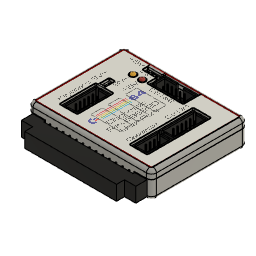
Diag_UP_PCB_v3_noVM v12 (Autodesk Fusion 360 design; units mm, degrees)
Autodesk Fusion 360 part; units mm, degrees
(part 1 of 2)
sketch "C64_Userport_Test" plane through (0, 0, 0) normal (0, 0, 1) x (1, 0, 0)
  line L0 (15.7163, 51.435) -> (15.7163, 52.705)
  line L1 (8.7313, 50.8) -> (8.0962, 51.435)
  line L2 (15.0813, 50.8) -> (15.7163, 51.435)
  line L3 (8.0962, 52.705) -> (8.7313, 53.34)
  line L4 (10.6363, 51.435) -> (10.0013, 50.8)
  line L5 (15.0813, 50.8) -> (13.8113, 50.8)
  line L6 (12.5412, 50.8) -> (11.2713, 50.8)
  line L7 (13.8113, 50.8) -> (13.1763, 51.435)
  line L8 (13.8113, 53.34) -> (15.0813, 53.34)
  line L9 (3.175, 30.6388) -> (2.54, 31.2738)
  line L10 (2.54, 33.8137) -> (2.54, 35.0838)
  line L11 (3.175, 33.1788) -> (2.54, 33.8137)
  line L12 (10.6363, 52.705) -> (11.2713, 53.34)
  line L13 (5.08, 32.5438) -> (5.08, 31.2738)
  arc A0 (8.3, 43.5) -> (8.3, 46.5) centre (7.5, 45) ccw
  line L14 (5.08, 35.0838) -> (5.08, 33.8137)
  line L15 (3.175, 35.7188) -> (2.54, 35.7188)
  line L16 (2.54, 31.2738) -> (2.54, 32.5438)
  arc A1 (6.7, 46.5) -> (6.7, 43.5) centre (7.5, 45) ccw
  arc A2 (6.7, 46.5) -> (6.7, 43.5) centre (7.5, 45) ccw
  line L17 (10.6363, 51.435) -> (10.6363, 52.705)
  line L18 (12.5412, 53.34) -> (13.1763, 52.705)
  line L19 (8.7313, 53.34) -> (10.0013, 53.34)
  line L20 (4.445, 30.6388) -> (3.175, 30.6388)
  line L21 (5.08, 35.0838) -> (4.445, 35.7188)
  line L22 (10.0013, 53.34) -> (10.6363, 52.705)
  line L23 (4.445, 33.1788) -> (3.175, 33.1788)
  line L24 (15.7163, 52.705) -> (15.7163, 53.34)
  line L25 (13.1763, 52.705) -> (13.8113, 53.34)
  line L26 (13.1763, 51.435) -> (12.5412, 50.8)
  line L27 (11.2713, 53.34) -> (12.5412, 53.34)
  line L28 (8.0962, 51.435) -> (8.0962, 52.705)
  line L29 (15.7163, 53.34) -> (15.0813, 53.34)
  line L30 (4.445, 33.1788) -> (5.08, 32.5438)
  line L31 (2.54, 35.7188) -> (2.54, 35.0838)
  line L32 (11.2713, 50.8) -> (10.6363, 51.435)
  line L33 (10.0013, 50.8) -> (8.7313, 50.8)
  line L34 (2.54, 32.5438) -> (3.175, 33.1788)
  arc A3 (13.8, 43.5) -> (13.8, 46.5) centre (13, 45) ccw
  arc A4 (13.8, 43.5) -> (13.8, 46.5) centre (13, 45) ccw
  arc A5 (8.3, 43.5) -> (8.3, 46.5) centre (7.5, 45) ccw
  line L35 (5.08, 31.2738) -> (4.445, 30.6388)
  line L36 (4.445, 35.7188) -> (3.175, 35.7188)
  line L37 (5.08, 33.8137) -> (4.445, 33.1788)
  line L38 (13.1763, 51.435) -> (13.1763, 52.705)
  arc A6 (12.2, 46.5) -> (12.2, 43.5) centre (13, 45) ccw
  arc A7 (12.2, 46.5) -> (12.2, 43.5) centre (13, 45) ccw
  arc A8 (15.9068, 14.224) -> (15.9068, 16.256) centre (15.9068, 15.24) ccw
  arc A9 (15.9068, 34.8615) -> (15.9068, 36.8935) centre (15.9068, 35.8775) ccw
  line L39 (32.6707, 38.7985) -> (32.6707, 32.9565)
  line L40 (15.9068, 32.9565) -> (15.9068, 34.8615)
  line L41 (32.6707, 18.161) -> (32.6707, 12.319)
  arc A10 (15.9068, 24.5427) -> (15.9068, 26.5747) centre (15.9068, 25.5587) ccw
  line L42 (32.6707, 38.7985) -> (15.9068, 38.7985)
  line L43 (15.9068, 18.161) -> (15.9068, 16.256)
  line L44 (15.9068, 32.9565) -> (32.6707, 32.9565)
  line L45 (15.9068, 22.6378) -> (15.9068, 24.5428)
  line L46 (32.6707, 28.4798) -> (32.6707, 22.6378)
  line L47 (15.9068, 28.4798) -> (15.9068, 26.5748)
  line L48 (15.9068, 22.6378) -> (32.6707, 22.6378)
  line L49 (15.9068, 12.319) -> (15.9068, 14.224)
  line L50 (15.9068, 12.319) -> (32.6707, 12.319)
  line L51 (15.9068, 38.7985) -> (15.9068, 36.8935)
  line L52 (32.6707, 28.4798) -> (15.9068, 28.4798)
  line L53 (32.6707, 18.161) -> (15.9068, 18.161)
  line L54 (9.6203, 51.816) -> (9.6203, 52.324)
  arc A11 (6.7, 43.5) -> (8.3, 43.5) centre (7.5, 45) ccw
  line L55 (11.6523, 51.816) -> (12.1603, 51.816)
  line L56 (4.064, 34.7028) -> (3.556, 34.7028)
  line L57 (14.1923, 51.816) -> (14.7003, 51.816)
  line L58 (9.1123, 51.816) -> (9.6203, 51.816)
  line L59 (4.064, 32.1628) -> (3.556, 32.1628)
  line L60 (12.1603, 52.324) -> (11.6523, 52.324)
  line L61 (4.064, 34.1948) -> (4.064, 34.7028)
  line L62 (3.556, 34.7028) -> (3.556, 34.1948)
  line L63 (14.7003, 52.324) -> (14.1923, 52.324)
  line L64 (3.556, 31.6548) -> (4.064, 31.6548)
  line L65 (14.1923, 52.324) -> (14.1923, 51.816)
  line L66 (14.7003, 51.816) -> (14.7003, 52.324)
  line L67 (3.556, 32.1628) -> (3.556, 31.6548)
  line L68 (3.556, 34.1948) -> (4.064, 34.1948)
  line L69 (9.1123, 52.324) -> (9.1123, 51.816)
  circle A12 centre (7.5, 45) radius 1.5
  line L70 (12.1603, 51.816) -> (12.1603, 52.324)
  line L71 (9.6203, 52.324) -> (9.1123, 52.324)
  line L72 (6.7, 46.5) -> (8.3, 46.5)
  line L73 (12.2, 46.5) -> (13.8, 46.5)
  line L74 (4.064, 31.6548) -> (4.064, 32.1628)
  line L75 (11.6523, 52.324) -> (11.6523, 51.816)
  arc A13 (12.2, 43.5) -> (13.8, 43.5) centre (13, 45) ccw
  circle A14 centre (13, 45) radius 1.5
sketch "DXF import" plane through (0, 0, 0) normal (0, 0, 1) x (1, 0, 0) in component "PCB"
  arc A0 (0, 1) -> (1, 0) centre (1, 1) ccw
  line L0 (53, 1) -> (53, 54)
  line L1 (0, 1) -> (0, 54)
  arc A1 (53, 54) -> (52, 55) centre (52, 54) ccw
  line L2 (52, 55) -> (1, 55)
  line L3 (1, 0) -> (52, 0)
  arc A2 (1, 55) -> (0, 54) centre (1, 54) ccw
  arc A3 (52, 0) -> (53, 1) centre (52, 1) ccw
  circle A4 centre (4, 51) radius 3.1
  line L4 (32.6707, 38.7985) -> (32.6707, 32.9565)
  arc A5 (15.9068, 24.5428) -> (15.9068, 26.5748) centre (15.9068, 25.5588) ccw
  line L5 (15.9068, 28.4798) -> (15.9068, 26.5748)
  line L6 (15.9068, 32.9565) -> (32.6707, 32.9565)
  line L7 (15.9068, 22.6378) -> (15.9068, 24.5428)
  line L8 (15.9068, 22.6378) -> (32.6707, 22.6378)
  line L9 (32.6707, 28.4798) -> (32.6707, 22.6378)
  line L10 (32.6707, 28.4798) -> (15.9068, 28.4798)
  line L11 (50.18, 0) -> (50.18, -1)
  line L12 (32.6707, 38.7985) -> (15.9068, 38.7985)
  circle A6 centre (49, 51) radius 3.1
  line L13 (15.9068, 18.161) -> (15.9068, 16.256)
  line L14 (46.72, -1) -> (46.72, 0)
  line L15 (15.9068, 12.319) -> (15.9068, 14.224)
  circle A7 centre (49, 51) radius 1.5875
  line L16 (46.72, 0) -> (46.22, 0)
  line L17 (32.6707, 18.161) -> (15.9068, 18.161)
  arc A8 (15.9068, 14.224) -> (15.9068, 16.256) centre (15.9068, 15.24) ccw
  line L18 (15.9068, 12.319) -> (32.6707, 12.319)
  line L19 (32.6707, 18.161) -> (32.6707, 12.319)
  line L20 (49.45, 0.1) -> (49.45, -1)
  line L21 (47.45, 0.1) -> (47.45, -1)
  line L22 (46.22, 0) -> (46.22, -1)
  line L23 (50.68, -1) -> (50.68, 0)
  arc A9 (15.9068, 34.8615) -> (15.9068, 36.8935) centre (15.9068, 35.8775) ccw
  line L24 (50.68, 0) -> (50.18, 0)
  line L25 (31.61, 0.1) -> (31.61, -1)
  line L26 (15.9068, 38.7985) -> (15.9068, 36.8935)
  circle A10 centre (4, 51) radius 1.5875
  line L27 (15.9068, 32.9565) -> (15.9068, 34.8615)
  line L28 (22.96, 0) -> (22.46, 0)
  line L29 (7.85, 0.1) -> (7.85, -1)
  line L30 (42.76, -1) -> (42.76, 0)
  line L31 (43.49, 0.1) -> (43.49, -1)
  line L32 (45.49, 0.1) -> (45.49, -1)
  line L33 (30.88, -1) -> (30.88, 0)
  line L34 (7.12, -1) -> (7.12, 0)
  line L35 (22.46, 0) -> (22.46, -1)
  line L36 (7.12, 0) -> (6.62, 0)
  line L37 (35.57, 0.1) -> (35.57, -1)
  line L38 (6.62, 0) -> (6.62, -1)
  line L39 (14.54, 0) -> (14.54, -1)
  line L40 (37.57, 0.1) -> (37.57, -1)
  line L41 (38.8, -1) -> (38.8, 0)
  line L42 (15.04, 0) -> (14.54, 0)
  line L43 (18.5, 0) -> (18.5, -1)
  line L44 (29.65, 0.1) -> (29.65, -1)
  line L45 (30.88, 0) -> (30.38, 0)
  line L46 (27.65, 0.1) -> (27.65, -1)
  line L47 (26.42, 0) -> (26.42, -1)
  line L48 (38.8, 0) -> (38.3, 0)
  line L49 (34.84, 0) -> (34.34, 0)
  line L50 (39.53, 0.1) -> (39.53, -1)
  line L51 (42.26, 0) -> (42.26, -1)
  line L52 (42.76, 0) -> (42.26, 0)
  line L53 (26.92, -1) -> (26.92, 0)
  line L54 (38.3, 0) -> (38.3, -1)
  line L55 (33.61, 0.1) -> (33.61, -1)
  line L56 (34.34, 0) -> (34.34, -1)
  line L57 (26.92, 0) -> (26.42, 0)
  line L58 (30.38, 0) -> (30.38, -1)
  line L59 (34.84, -1) -> (34.84, 0)
  line L60 (41.53, 0.1) -> (41.53, -1)
  line L61 (21.73, 0.1) -> (21.73, -1)
  line L62 (15.77, 0.1) -> (15.77, -1)
  line L63 (11.08, -1) -> (11.08, 0)
  line L64 (23.69, 0.1) -> (23.69, -1)
  line L65 (19.73, 0.1) -> (19.73, -1)
  line L66 (25.69, 0.1) -> (25.69, -1)
  line L67 (19, -1) -> (19, 0)
  line L68 (11.81, 0.1) -> (11.81, -1)
  line L69 (54.17, -6.8) -> (54.17, -11.6)
  line L70 (11.08, 0) -> (10.58, 0)
  line L71 (22.96, -1) -> (22.96, 0)
  line L72 (55.97, -6.8) -> (54.17, -6.8)
  line L73 (-6.03, -6.8) -> (-7.58, -6.8)
  line L74 (59.37, -6.8) -> (55.97, -6.8)
  line L75 (60.92, -6.8) -> (59.37, -6.8)
  line L76 (19, 0) -> (18.5, 0)
  line L77 (9.85, 0.1) -> (9.85, -1)
  line L78 (53.47, 0) -> (53.47, -1)
  line L79 (3.16, -1) -> (3.16, 0)
  line L80 (17.77, 0.1) -> (17.77, -1)
  line L81 (-2.63, -6.8) -> (-2.63, -5.2)
  line L82 (-4.33, 0) -> (-4.33, -2.8667)
  line L83 (57.67, -3.6853) -> (57.67, -3.548)
  line L84 (55.97, -4.2) -> (55.97, -2.6)
  line L85 (59.37, -1.6) -> (59.37, 0)
  line L86 (60.92, 0) -> (59.37, 0)
  line L87 (59.37, 0) -> (57.67, 0)
  line L88 (-4.33, -3.548) -> (-4.33, -3.6853)
  line L89 (-4.33, -4.3667) -> (-4.33, -7.2333)
  line L90 (55.97, -1.6) -> (55.97, 0)
  line L91 (57.67, 0) -> (55.97, 0)
  line L92 (-0.83, -6.8) -> (-2.63, -6.8)
  line L93 (-2.63, -4.2) -> (-2.63, -2.6)
  line L94 (-4.33, -8.7333) -> (-4.33, -11.6)
  line L95 (-4.33, 0) -> (-6.03, 0)
  line L96 (10.58, 0) -> (10.58, -1)
  line L97 (13.81, 0.1) -> (13.81, -1)
  line L98 (5.89, 0.1) -> (5.89, -1)
  line L99 (-2.63, -1.6) -> (-2.63, 0)
  line L100 (-6.03, -1.6) -> (-6.03, 0)
  line L101 (55.97, 0) -> (53.47, 0)
  line L102 (-7.58, 0) -> (-7.58, -6.8)
  line L103 (3.16, 0) -> (2.66, 0)
  line L104 (3.89, 0.1) -> (3.89, -1)
  line L105 (15.04, -1) -> (15.04, 0)
  line L106 (59.37, -4.2) -> (59.37, -2.6)
  line L107 (-6.03, -6.8) -> (-6.03, -5.2)
  line L108 (2.66, 0) -> (2.66, -1)
  line L109 (51.81, 14.73) -> (52.6038, 14.73)
  line L110 (52.6038, 23.62) -> (52.6038, 17.27)
  line L111 (-0.13, 0) -> (-2.63, 0)
  line L112 (60.92, 0) -> (60.92, -6.8)
  line L113 (46.2537, 8.38) -> (44.825, 8.38)
  line L114 (51.81, 17.27) -> (52.6038, 17.27)
  line L115 (-0.83, -11.6) -> (-0.83, -6.8)
  line L116 (-6.03, 0) -> (-7.58, 0)
  line L117 (57.67, -2.8667) -> (57.67, 0)
  line L118 (51.3338, 17.27) -> (51.81, 17.27)
  line L119 (46.2537, 23.62) -> (52.6038, 23.62)
  line L120 (44.6662, 22.35) -> (44.825, 22.35)
  line L121 (51.3338, 9.65) -> (46.2537, 9.65)
  line L122 (44.825, 22.35) -> (44.825, 22.8263)
  line L123 (57.67, -11.6) -> (57.67, -8.7333)
  line L124 (43.3962, 23.62) -> (44.825, 23.62)
  line L125 (51.81, 14.73) -> (51.81, 9.1737)
  line L126 (46.2537, 22.35) -> (46.2537, 22.8263)
  line L127 (57.67, -7.2333) -> (57.67, -4.3667)
  line L128 (44.825, 8.38) -> (43.3962, 8.38)
  line L129 (51.3338, 22.35) -> (51.3338, 17.27)
  line L130 (44.825, 9.65) -> (44.825, 9.1737)
  line L131 (55.97, -6.8) -> (55.97, -5.2)
  line L132 (51.3338, 22.35) -> (51.81, 22.8263)
  line L133 (51.3338, 14.73) -> (51.3338, 9.65)
  line L134 (-4.33, -7.9147) -> (-4.33, -8.052)
  line L135 (53.47, -1) -> (-0.13, -1)
  line L136 (-2.63, -6.8) -> (-6.03, -6.8)
  line L137 (44.6662, 9.65) -> (44.6662, 22.35)
  line L138 (46.2537, 22.35) -> (51.3338, 22.35)
  line L139 (54.17, -11.6) -> (-0.83, -11.6)
  line L140 (57.67, -8.052) -> (57.67, -7.9147)
  line L141 (52.6038, 14.73) -> (52.6038, 8.38)
  line L142 (51.3338, 17.27) -> (51.3338, 14.73)
  line L143 (43.3962, 8.38) -> (43.3962, 23.62)
  line L144 (46.2537, 9.65) -> (44.825, 9.65)
  line L145 (51.3338, 14.73) -> (51.81, 14.73)
  line L146 (-6.03, -4.2) -> (-6.03, -2.6)
  line L147 (52.6038, 17.27) -> (52.6038, 14.73)
  line L148 (52.6038, 8.38) -> (46.2537, 8.38)
  line L149 (44.825, 9.65) -> (44.6662, 9.65)
  line L150 (59.37, -6.8) -> (59.37, -5.2)
  line L151 (44.825, 23.62) -> (46.2537, 23.62)
  line L152 (44.825, 22.35) -> (46.2537, 22.35)
  line L153 (-2.63, 0) -> (-4.33, 0)
  line L154 (-0.13, -1) -> (-0.13, 0)
  arc A11 (43.3962, 35.4763) -> (43.3962, 34.3651) centre (43.3962, 34.9207) ccw
  line L155 (46.2537, 9.1737) -> (51.81, 9.1737)
  line L156 (44.19, 9.1737) -> (44.6662, 9.65)
  arc A12 (43.3962, 10.92) -> (43.3962, 9.65) centre (43.3962, 10.285) ccw
  line L157 (44.825, 22.8263) -> (44.19, 22.8263)
  arc A13 (43.3962, 27.38) -> (43.3962, 26.11) centre (43.3962, 26.745) ccw
  line L158 (44.825, 24.84) -> (43.3962, 24.84)
  line L159 (44.825, 25.6337) -> (44.825, 24.84)
  line L160 (51.81, 25.6337) -> (51.3338, 26.11)
  arc A14 (43.3962, 22.35) -> (43.3962, 21.08) centre (43.3962, 21.715) ccw
  line L161 (44.19, 25.6337) -> (44.825, 25.6337)
  line L162 (44.6662, 26.11) -> (44.6662, 43.89)
  line L163 (44.825, 26.11) -> (44.6662, 26.11)
  line L164 (43.3962, 45.16) -> (44.825, 45.16)
  line L165 (46.2537, 44.3663) -> (46.2537, 45.16)
  line L166 (44.825, 43.89) -> (44.825, 44.3663)
  line L167 (51.81, 9.1737) -> (51.3338, 9.65)
  arc A15 (43.3962, 16.4763) -> (43.3962, 15.3651) centre (43.3962, 15.9207) ccw
  line L168 (46.2537, 22.8263) -> (46.2537, 23.62)
  line L169 (44.19, 9.1737) -> (44.825, 9.1737)
  line L170 (44.825, 9.1737) -> (44.825, 8.38)
  line L171 (51.81, 17.27) -> (51.81, 22.8263)
  line L172 (46.2537, 9.65) -> (46.2537, 9.1737)
  line L173 (46.2537, 22.8263) -> (51.81, 22.8263)
  line L174 (44.6662, 22.35) -> (44.19, 22.8263)
  line L175 (51.3338, 37.0638) -> (51.3338, 32.9362)
  line L176 (51.3338, 37.0638) -> (51.81, 37.0638)
  line L177 (44.825, 44.3663) -> (44.19, 44.3663)
  line L178 (51.3338, 43.89) -> (51.81, 44.3663)
  line L179 (44.825, 43.89) -> (46.2537, 43.89)
  line L180 (46.2537, 25.6337) -> (46.2537, 24.84)
  line L181 (51.3338, 43.89) -> (51.3338, 37.0638)
  line L182 (46.2537, 43.89) -> (46.2537, 44.3663)
  line L183 (51.81, 32.9362) -> (52.6038, 32.9362)
  line L184 (51.3338, 26.11) -> (46.2537, 26.11)
  line L185 (46.2537, 9.1737) -> (46.2537, 8.38)
  line L186 (44.19, 25.6337) -> (44.19, 44.3663)
  line L187 (44.19, 9.1737) -> (44.19, 22.8263)
  line L188 (46.2537, 25.6337) -> (51.81, 25.6337)
  line L189 (44.19, 25.6337) -> (44.6662, 26.11)
  line L190 (44.825, 22.8263) -> (44.825, 23.62)
  line L191 (51.81, 32.9362) -> (51.81, 25.6337)
  line L192 (44.6662, 43.89) -> (44.825, 43.89)
  arc A16 (43.3962, 43.89) -> (43.3962, 42.62) centre (43.3962, 43.255) ccw
  line L193 (44.825, 26.11) -> (44.825, 25.6337)
  line L194 (52.6038, 37.0638) -> (52.6038, 32.9362)
  line L195 (43.3962, 24.84) -> (43.3962, 45.16)
  line L196 (46.2537, 26.11) -> (44.825, 26.11)
  line L197 (44.825, 44.3663) -> (44.825, 45.16)
  line L198 (37.16, 46.825) -> (37.16, 45.3962)
  line L199 (18.11, 48.2537) -> (17.6337, 48.2537)
  line L200 (37.16, 54.6038) -> (37.16, 48.2537)
  arc A17 (26.5238, 45.3962) -> (27.635, 45.3962) centre (27.0794, 45.3962) ccw
  line L201 (51.3338, 32.9362) -> (51.3338, 26.11)
  line L202 (36.3663, 46.19) -> (36.3663, 46.825)
  line L203 (51.81, 37.0638) -> (51.81, 44.3663)
  line L204 (29.0638, 53.81) -> (29.0638, 54.6038)
  line L205 (29.0638, 53.3338) -> (35.89, 53.3338)
  line L206 (46.2537, 45.16) -> (52.6038, 45.16)
  line L207 (17.6337, 46.825) -> (16.84, 46.825)
  line L208 (37.16, 48.2537) -> (37.16, 46.825)
  line L209 (46.2537, 43.89) -> (51.3338, 43.89)
  line L210 (52.6038, 32.9362) -> (52.6038, 24.84)
  line L211 (18.11, 53.3338) -> (24.9362, 53.3338)
  line L212 (36.3663, 48.2537) -> (36.3663, 53.81)
  line L213 (52.6038, 45.16) -> (52.6038, 37.0638)
  line L214 (51.3338, 32.9362) -> (51.81, 32.9362)
  line L215 (44.6662, 43.89) -> (44.19, 44.3663)
  line L216 (17.6337, 46.825) -> (17.6337, 46.19)
  line L217 (18.11, 46.6662) -> (18.11, 46.825)
  line L218 (52.6038, 24.84) -> (46.2537, 24.84)
  line L219 (18.11, 46.825) -> (18.11, 48.2537)
  line L220 (24.9362, 53.81) -> (24.9362, 54.6038)
  line L221 (29.0638, 54.6038) -> (37.16, 54.6038)
  line L222 (29.0638, 53.3338) -> (29.0638, 53.81)
  line L223 (18.11, 46.825) -> (17.6337, 46.825)
  line L224 (36.3663, 46.19) -> (17.6337, 46.19)
  line L225 (46.2537, 44.3663) -> (51.81, 44.3663)
  line L226 (29.0638, 53.81) -> (36.3663, 53.81)
  line L227 (18.11, 53.3338) -> (17.6337, 53.81)
  line L228 (44.825, 45.16) -> (46.2537, 45.16)
  line L229 (46.2537, 24.84) -> (44.825, 24.84)
  arc A18 (18.11, 45.3962) -> (19.38, 45.3962) centre (18.745, 45.3962) ccw
  line L230 (24.9362, 53.3338) -> (29.0638, 53.3338)
  line L231 (46.2537, 26.11) -> (46.2537, 25.6337)
  line L232 (18.11, 46.6662) -> (17.6337, 46.19)
  line L233 (36.3663, 46.19) -> (35.89, 46.6662)
  line L234 (51.81, 37.0638) -> (52.6038, 37.0638)
  line L235 (35.89, 48.2537) -> (35.89, 46.825)
  line L236 (2.6987, 27.4638) -> (2.8575, 27.4638)
  line L237 (16.84, 46.825) -> (16.84, 48.2537)
  line L238 (9.3663, 9.6837) -> (4.2862, 9.6837)
  line L239 (9.8425, 20.6376) -> (9.8425, 27.9401)
  line L240 (18.11, 48.2537) -> (18.11, 53.3338)
  line L241 (4.2862, 28.7338) -> (10.6363, 28.7338)
  line L242 (9.3663, 16.5099) -> (9.3663, 9.6837)
  arc A19 (1.4287, 27.4638) -> (1.4287, 26.1938) centre (1.4287, 26.8288) ccw
  line L243 (10.6363, 28.7338) -> (10.6363, 20.6376)
  line L244 (2.8575, 9.6837) -> (2.6987, 9.6837)
  line L245 (24.9362, 53.3338) -> (24.9362, 53.81)
  arc A20 (34.62, 45.3962) -> (35.89, 45.3962) centre (35.255, 45.3962) ccw
  line L246 (9.3663, 20.6376) -> (9.3663, 16.5099)
  line L247 (17.6337, 48.2537) -> (16.84, 48.2537)
  line L248 (24.9362, 53.81) -> (17.6337, 53.81)
  line L249 (2.6987, 27.4638) -> (2.2225, 27.9401)
  line L250 (4.2862, 9.6837) -> (4.2862, 9.2074)
  line L251 (36.3663, 46.825) -> (37.16, 46.825)
  line L252 (16.84, 54.6038) -> (24.9362, 54.6038)
  line L253 (35.89, 48.2537) -> (36.3663, 48.2537)
  line L254 (17.6337, 48.2537) -> (17.6337, 53.81)
  line L255 (16.84, 45.3962) -> (16.84, 46.825)
  line L256 (35.89, 53.3338) -> (35.89, 48.2537)
  line L257 (10.6363, 20.6376) -> (10.6363, 16.5099)
  line L258 (2.8575, 28.7338) -> (4.2862, 28.7338)
  line L259 (35.89, 46.6662) -> (18.11, 46.6662)
  line L260 (24.9362, 54.6038) -> (29.0638, 54.6038)
  line L261 (1.4287, 28.7338) -> (2.8575, 28.7338)
  line L262 (35.89, 46.825) -> (36.3663, 46.825)
  line L263 (36.3663, 48.2537) -> (37.16, 48.2537)
  line L264 (35.89, 46.825) -> (35.89, 46.6662)
  line L265 (2.8575, 8.4138) -> (1.4287, 8.4138)
  line L266 (1.4287, 8.4138) -> (1.4287, 28.7338)
  line L267 (37.16, 45.3962) -> (16.84, 45.3962)
  line L268 (10.6363, 16.5099) -> (10.6363, 8.4138)
  line L269 (4.2862, 27.9401) -> (4.2862, 28.7338)
  arc A21 (1.4287, 10.9537) -> (1.4287, 9.6837) centre (1.4287, 10.3187) ccw
  line L270 (9.3663, 20.6376) -> (9.8425, 20.6376)
  line L271 (36.3663, 53.81) -> (35.89, 53.3338)
  line L272 (2.8575, 27.9401) -> (2.2225, 27.9401)
  line L273 (9.3663, 16.5099) -> (9.8425, 16.5099)
  line L274 (2.8575, 9.6837) -> (2.8575, 9.2074)
  line L275 (2.2225, 9.2074) -> (2.6987, 9.6837)
  arc A22 (1.4287, 19.05) -> (1.4287, 17.9388) centre (1.4287, 18.4944) ccw
  line L276 (16.84, 48.2537) -> (16.84, 54.6038)
  line L277 (4.2862, 27.4638) -> (9.3663, 27.4638)
  line L278 (4.2862, 9.2074) -> (9.8425, 9.2074)
  line L279 (2.8575, 9.2074) -> (2.8575, 8.4138)
  line L280 (9.8425, 16.5099) -> (9.8425, 9.2074)
  line L281 (10.6363, 8.4138) -> (4.2862, 8.4138)
  line L282 (9.8425, 20.6376) -> (10.6363, 20.6376)
  line L283 (9.3663, 27.4638) -> (9.3663, 20.6376)
  line L284 (2.2225, 9.2074) -> (2.2225, 27.9401)
  line L285 (2.8575, 27.4638) -> (4.2862, 27.4638)
  line L286 (2.8575, 27.4638) -> (2.8575, 27.9401)
  line L287 (2.6987, 9.6837) -> (2.6987, 27.4638)
  line L288 (2.2225, 9.2074) -> (2.8575, 9.2074)
  line L289 (9.8425, 9.2074) -> (9.3663, 9.6837)
  line L290 (9.8425, 16.5099) -> (10.6363, 16.5099)
  line L291 (4.2862, 8.4138) -> (2.8575, 8.4138)
  line L292 (2.8575, 27.9401) -> (2.8575, 28.7338)
  line L293 (4.2862, 9.2074) -> (4.2862, 8.4138)
  line L294 (4.2862, 27.9401) -> (9.8425, 27.9401)
  line L295 (9.3663, 27.4638) -> (9.8425, 27.9401)
  line L296 (4.2862, 27.4638) -> (4.2862, 27.9401)
  line L297 (4.2862, 9.6837) -> (2.8575, 9.6837)
  line L298 (52, 0) -> (59.45, 0)
  line L299 (27.254, 51.016) -> (27.254, 51.524)
  line L300 (24.206, 48.476) -> (24.714, 48.476)
  line L301 (26.746, 48.984) -> (26.746, 48.476)
  line L302 (32.334, 48.984) -> (31.826, 48.984)
  line L303 (32.334, 51.524) -> (31.826, 51.524)
  line L304 (26.746, 48.476) -> (27.254, 48.476)
  line L305 (24.714, 51.016) -> (24.714, 51.524)
  line L306 (21.666, 48.984) -> (21.666, 48.476)
  line L307 (21.666, 48.476) -> (22.174, 48.476)
  line L308 (31.826, 48.476) -> (32.334, 48.476)
  line L309 (24.714, 48.476) -> (24.714, 48.984)
  line L310 (21.666, 51.524) -> (21.666, 51.016)
  line L311 (27.254, 48.476) -> (27.254, 48.984)
  line L312 (24.206, 51.016) -> (24.714, 51.016)
  line L313 (29.794, 51.524) -> (29.286, 51.524)
  line L314 (21.666, 51.016) -> (22.174, 51.016)
  line L315 (24.206, 48.984) -> (24.206, 48.476)
  line L316 (27.254, 51.524) -> (26.746, 51.524)
  line L317 (29.286, 51.524) -> (29.286, 51.016)
  line L318 (22.174, 48.984) -> (21.666, 48.984)
  line L319 (31.826, 51.524) -> (31.826, 51.016)
  line L320 (29.286, 48.984) -> (29.286, 48.476)
  line L321 (29.286, 51.016) -> (29.794, 51.016)
  line L322 (26.746, 51.524) -> (26.746, 51.016)
  line L323 (32.334, 48.476) -> (32.334, 48.984)
  line L324 (22.174, 51.524) -> (21.666, 51.524)
  line L325 (29.794, 48.476) -> (29.794, 48.984)
  line L326 (49.016, 32.206) -> (49.524, 32.206)
  line L327 (31.826, 51.016) -> (32.334, 51.016)
  line L328 (24.206, 51.524) -> (24.206, 51.016)
  line L329 (29.794, 51.016) -> (29.794, 51.524)
  line L330 (31.826, 48.984) -> (31.826, 48.476)
  line L331 (22.174, 51.016) -> (22.174, 51.524)
  line L332 (32.334, 51.016) -> (32.334, 51.524)
  line L333 (29.286, 48.476) -> (29.794, 48.476)
  line L334 (27.254, 48.984) -> (26.746, 48.984)
  line L335 (22.174, 48.476) -> (22.174, 48.984)
  line L336 (24.714, 51.524) -> (24.206, 51.524)
  line L337 (26.746, 51.016) -> (27.254, 51.016)
  line L338 (24.714, 48.984) -> (24.206, 48.984)
  line L339 (29.794, 48.984) -> (29.286, 48.984)
  line L340 (5.0165, 15.7798) -> (5.0165, 16.2878)
  line L341 (7.5565, 16.2878) -> (7.0485, 16.2878)
  line L342 (7.5565, 20.8597) -> (7.5565, 21.3677)
  line L343 (7.0485, 18.8278) -> (7.0485, 18.3198)
  line L344 (5.0165, 23.3998) -> (5.0165, 23.9078)
  line L345 (5.0165, 13.7478) -> (4.5085, 13.7478)
  line L346 (7.0485, 20.8597) -> (7.5565, 20.8597)
  line L347 (7.0485, 13.2398) -> (7.5565, 13.2398)
  line L348 (5.0165, 20.8597) -> (5.0165, 21.3677)
  line L349 (5.0165, 18.3198) -> (5.0165, 18.8278)
  line L350 (4.5085, 15.7798) -> (5.0165, 15.7798)
  line L351 (5.0165, 16.2878) -> (4.5085, 16.2878)
  line L352 (5.0165, 13.2398) -> (5.0165, 13.7478)
  line L353 (5.0165, 18.8278) -> (4.5085, 18.8278)
  line L354 (7.0485, 16.2878) -> (7.0485, 15.7798)
  line L355 (7.5565, 18.3198) -> (7.5565, 18.8278)
  line L356 (4.5085, 18.8278) -> (4.5085, 18.3198)
  line L357 (7.5565, 13.7478) -> (7.0485, 13.7478)
  line L358 (7.0485, 21.3677) -> (7.0485, 20.8597)
  line L359 (7.0485, 18.3198) -> (7.5565, 18.3198)
  line L360 (4.5085, 16.2878) -> (4.5085, 15.7798)
  line L361 (4.5085, 13.7478) -> (4.5085, 13.2398)
  line L362 (7.0485, 15.7798) -> (7.5565, 15.7798)
  line L363 (4.5085, 18.3198) -> (5.0165, 18.3198)
  line L364 (7.5565, 15.7798) -> (7.5565, 16.2878)
  line L365 (7.5565, 18.8278) -> (7.0485, 18.8278)
  line L366 (4.5085, 20.8597) -> (5.0165, 20.8597)
  line L367 (7.5565, 13.2398) -> (7.5565, 13.7478)
  line L368 (7.5565, 21.3677) -> (7.0485, 21.3677)
  line L369 (7.0485, 13.7478) -> (7.0485, 13.2398)
  line L370 (4.5085, 21.3677) -> (4.5085, 20.8597)
  line L371 (7.0485, 23.3998) -> (7.5565, 23.3998)
  line L372 (45.49, 0.1) -> (45.49, 4)
  line L373 (49.45, 0.1) -> (49.45, 4)
  line L374 (47.95, 3) -> (47.95, 2)
  line L375 (35.57, 0.1) -> (35.57, 4)
  line L376 (7.5565, 23.9078) -> (7.0485, 23.9078)
  line L377 (48.95, 3) -> (48.95, 2)
  line L378 (4.5085, 13.2398) -> (5.0165, 13.2398)
  line L379 (7.5565, 23.3998) -> (7.5565, 23.9078)
  arc A23 (49.45, 4) -> (47.45, 4) centre (48.45, 4) ccw
  line L380 (47.45, 0.1) -> (47.45, 4)
  line L381 (5.0165, 21.3677) -> (4.5085, 21.3677)
  arc A24 (48.95, 3) -> (47.95, 3) centre (48.45, 3) ccw
  arc A25 (47.95, 2) -> (48.95, 2) centre (48.45, 2) ccw
  line L382 (4.5085, 23.9078) -> (4.5085, 23.3998)
  line L383 (7.0485, 23.9078) -> (7.0485, 23.3998)
  line L384 (5.0165, 23.9078) -> (4.5085, 23.9078)
  line L385 (4.5085, 23.3998) -> (5.0165, 23.3998)
  arc A26 (29.15, 3) -> (28.15, 3) centre (28.65, 3) ccw
  arc A27 (25.69, 4) -> (23.69, 4) centre (24.69, 4) ccw
  line L386 (37.07, 3) -> (37.07, 2)
  arc A28 (43.99, 2) -> (44.99, 2) centre (44.49, 2) ccw
  line L387 (43.99, 3) -> (43.99, 2)
  line L388 (32.11, 3) -> (32.11, 2)
  arc A29 (44.99, 3) -> (43.99, 3) centre (44.49, 3) ccw
  line L389 (43.49, 0.1) -> (43.49, 4)
  arc A30 (37.07, 3) -> (36.07, 3) centre (36.57, 3) ccw
  arc A31 (40.03, 2) -> (41.03, 2) centre (40.53, 2) ccw
  arc A32 (33.61, 4) -> (31.61, 4) centre (32.61, 4) ccw
  line L390 (40.03, 3) -> (40.03, 2)
  line L391 (25.69, 0.1) -> (25.69, 4)
  arc A33 (28.15, 2) -> (29.15, 2) centre (28.65, 2) ccw
  line L392 (31.61, 0.1) -> (31.61, 4)
  arc A34 (45.49, 4) -> (43.49, 4) centre (44.49, 4) ccw
  line L393 (29.15, 3) -> (29.15, 2)
  arc A35 (25.19, 3) -> (24.19, 3) centre (24.69, 3) ccw
  line L394 (44.99, 3) -> (44.99, 2)
  arc A36 (41.03, 3) -> (40.03, 3) centre (40.53, 3) ccw
  arc A37 (41.53, 4) -> (39.53, 4) centre (40.53, 4) ccw
  line L395 (23.69, 0.1) -> (23.69, 4)
  line L396 (36.07, 3) -> (36.07, 2)
  line L397 (37.57, 0.1) -> (37.57, 4)
  line L398 (41.03, 3) -> (41.03, 2)
  line L399 (27.65, 0.1) -> (27.65, 4)
  line L400 (25.19, 3) -> (25.19, 2)
  line L401 (28.15, 3) -> (28.15, 2)
  line L402 (29.65, 0.1) -> (29.65, 4)
  line L403 (33.61, 0.1) -> (33.61, 4)
  arc A38 (13.81, 4) -> (11.81, 4) centre (12.81, 4) ccw
  line L404 (5.89, 0.1) -> (5.89, 4)
  line L405 (21.23, 3) -> (21.23, 2)
  line L406 (8.35, 3) -> (8.35, 2)
  line L407 (21.73, 0.1) -> (21.73, 4)
  line L408 (9.85, 0.1) -> (9.85, 4)
  line L409 (13.81, 0.1) -> (13.81, 4)
  line L410 (13.31, 3) -> (13.31, 2)
  arc A39 (12.31, 2) -> (13.31, 2) centre (12.81, 2) ccw
  line L411 (3.89, 0.1) -> (3.89, 4)
  line L412 (4.39, 3) -> (4.39, 2)
  arc A40 (29.65, 4) -> (27.65, 4) centre (28.65, 4) ccw
  arc A41 (37.57, 4) -> (35.57, 4) centre (36.57, 4) ccw
  line L413 (19.73, 0.1) -> (19.73, 4)
  arc A42 (9.35, 3) -> (8.35, 3) centre (8.85, 3) ccw
  line L414 (41.53, 0.1) -> (41.53, 4)
  line L415 (11.81, 0.1) -> (11.81, 4)
  arc A43 (36.07, 2) -> (37.07, 2) centre (36.57, 2) ccw
  arc A44 (17.27, 3) -> (16.27, 3) centre (16.77, 3) ccw
  line L416 (33.11, 3) -> (33.11, 2)
  line L417 (15.77, 0.1) -> (15.77, 4)
  line L418 (20.23, 3) -> (20.23, 2)
  line L419 (17.27, 3) -> (17.27, 2)
  line L420 (9.35, 3) -> (9.35, 2)
  arc A45 (13.31, 3) -> (12.31, 3) centre (12.81, 3) ccw
  line L421 (17.77, 0.1) -> (17.77, 4)
  arc A46 (5.39, 3) -> (4.39, 3) centre (4.89, 3) ccw
  line L422 (12.31, 3) -> (12.31, 2)
  arc A47 (8.35, 2) -> (9.35, 2) centre (8.85, 2) ccw
  line L423 (5.39, 3) -> (5.39, 2)
  arc A48 (32.11, 2) -> (33.11, 2) centre (32.61, 2) ccw
  arc A49 (33.11, 3) -> (32.11, 3) centre (32.61, 3) ccw
  line L424 (39.53, 0.1) -> (39.53, 4)
  arc A50 (24.19, 2) -> (25.19, 2) centre (24.69, 2) ccw
  arc A51 (9.85, 4) -> (7.85, 4) centre (8.85, 4) ccw
  arc A52 (21.23, 3) -> (20.23, 3) centre (20.73, 3) ccw
  line L425 (49.524, 16.254) -> (49.016, 16.254)
  line L426 (46.984, 16.254) -> (46.476, 16.254)
  line L427 (49.016, 15.746) -> (49.524, 15.746)
  arc A53 (5.89, 4) -> (3.89, 4) centre (4.89, 4) ccw
  line L428 (46.984, 18.794) -> (46.476, 18.794)
  arc A54 (4.39, 2) -> (5.39, 2) centre (4.89, 2) ccw
  line L429 (46.476, 16.254) -> (46.476, 15.746)
  line L430 (49.016, 13.714) -> (49.016, 13.206)
  line L431 (7.85, 0.1) -> (7.85, 4)
  line L432 (49.524, 15.746) -> (49.524, 16.254)
  line L433 (49.524, 13.714) -> (49.016, 13.714)
  line L434 (16.27, 3) -> (16.27, 2)
  line L435 (46.984, 13.206) -> (46.984, 13.714)
  line L436 (24.19, 3) -> (24.19, 2)
  arc A55 (21.73, 4) -> (19.73, 4) centre (20.73, 4) ccw
  line L437 (46.476, 13.206) -> (46.984, 13.206)
  arc A56 (16.27, 2) -> (17.27, 2) centre (16.77, 2) ccw
  line L438 (46.476, 18.794) -> (46.476, 18.286)
  arc A57 (17.77, 4) -> (15.77, 4) centre (16.77, 4) ccw
  line L439 (46.984, 18.286) -> (46.984, 18.794)
  line L440 (46.476, 15.746) -> (46.984, 15.746)
  arc A58 (20.23, 2) -> (21.23, 2) centre (20.73, 2) ccw
  line L441 (46.984, 15.746) -> (46.984, 16.254)
  line L442 (49.016, 39.826) -> (49.524, 39.826)
  line L443 (49.524, 32.714) -> (49.016, 32.714)
  line L444 (46.984, 35.254) -> (46.476, 35.254)
  line L445 (49.524, 40.334) -> (49.016, 40.334)
  line L446 (46.476, 32.714) -> (46.476, 32.206)
  line L447 (46.476, 35.254) -> (46.476, 34.746)
  line L448 (49.016, 30.174) -> (49.016, 29.666)
  line L449 (49.016, 37.286) -> (49.524, 37.286)
  line L450 (46.476, 18.286) -> (46.984, 18.286)
  line L451 (49.016, 32.714) -> (49.016, 32.206)
  line L452 (46.476, 34.746) -> (46.984, 34.746)
  line L453 (46.476, 32.206) -> (46.984, 32.206)
  line L454 (49.524, 37.286) -> (49.524, 37.794)
  line L455 (46.984, 13.714) -> (46.476, 13.714)
  line L456 (49.016, 13.206) -> (49.524, 13.206)
  line L457 (46.476, 29.666) -> (46.984, 29.666)
  line L458 (49.016, 37.794) -> (49.016, 37.286)
  line L459 (49.524, 30.174) -> (49.016, 30.174)
  line L460 (49.016, 29.666) -> (49.524, 29.666)
  line L461 (49.524, 32.206) -> (49.524, 32.714)
  line L462 (46.476, 30.174) -> (46.476, 29.666)
  line L463 (46.984, 34.746) -> (46.984, 35.254)
  line L464 (46.476, 40.334) -> (46.476, 39.826)
  line L465 (46.476, 37.286) -> (46.984, 37.286)
  line L466 (49.016, 34.746) -> (49.524, 34.746)
  line L467 (46.476, 37.794) -> (46.476, 37.286)
  line L468 (46.984, 39.826) -> (46.984, 40.334)
  line L469 (46.984, 37.794) -> (46.476, 37.794)
  line L470 (49.524, 18.286) -> (49.524, 18.794)
  line L471 (49.524, 13.206) -> (49.524, 13.714)
  line L472 (49.016, 18.286) -> (49.524, 18.286)
  line L473 (49.524, 18.794) -> (49.016, 18.794)
  line L474 (49.016, 35.254) -> (49.016, 34.746)
  line L475 (46.476, 39.826) -> (46.984, 39.826)
  line L476 (46.984, 32.714) -> (46.476, 32.714)
  line L477 (49.524, 37.794) -> (49.016, 37.794)
  line L478 (46.476, 13.714) -> (46.476, 13.206)
  line L479 (49.524, 39.826) -> (49.524, 40.334)
  line L480 (46.984, 37.286) -> (46.984, 37.794)
  line L481 (49.524, 29.666) -> (49.524, 30.174)
  line L482 (49.016, 18.794) -> (49.016, 18.286)
  line L483 (49.016, 40.334) -> (49.016, 39.826)
  line L484 (46.984, 29.666) -> (46.984, 30.174)
  line L485 (46.984, 40.334) -> (46.476, 40.334)
  line L486 (49.016, 16.254) -> (49.016, 15.746)
  line L487 (46.984, 30.174) -> (46.476, 30.174)
  line L488 (49.524, 35.254) -> (49.016, 35.254)
  line L489 (49.524, 34.746) -> (49.524, 35.254)
  line L490 (46.984, 32.206) -> (46.984, 32.714)
  circle A59 centre (7.5, 45) radius 1.5
  arc A60 (6.7, 46.5) -> (6.7, 43.5) centre (7.5, 45) ccw
  arc A61 (6.7, 43.5) -> (8.3, 43.5) centre (7.5, 45) ccw
  arc A62 (8.3, 43.5) -> (8.3, 46.5) centre (7.5, 45) ccw
  line L491 (6.7, 46.5) -> (8.3, 46.5)
  arc A63 (12.2, 46.5) -> (12.2, 43.5) centre (13, 45) ccw
  line L492 (12.2, 46.5) -> (13.8, 46.5)
  circle A64 centre (13, 45) radius 1.5
  arc A65 (12.2, 43.5) -> (13.8, 43.5) centre (13, 45) ccw
  arc A66 (13.8, 43.5) -> (13.8, 46.5) centre (13, 45) ccw
  line L493 (8.7313, 53.34) -> (10.0013, 53.34)
  line L494 (8.0962, 52.705) -> (8.7313, 53.34)
  line L495 (8.0962, 51.435) -> (8.0962, 52.705)
  line L496 (8.7313, 50.8) -> (8.0962, 51.435)
  line L497 (10.0013, 50.8) -> (8.7313, 50.8)
  line L498 (10.6363, 51.435) -> (10.0013, 50.8)
  line L499 (9.1123, 51.816) -> (9.6203, 51.816)
  line L500 (9.1123, 52.324) -> (9.1123, 51.816)
  line L501 (9.6203, 52.324) -> (9.1123, 52.324)
  line L502 (9.6203, 51.816) -> (9.6203, 52.324)
  line L503 (10.0013, 53.34) -> (10.6363, 52.705)
  line L504 (10.6363, 51.435) -> (10.6363, 52.705)
  line L505 (11.2713, 50.8) -> (10.6363, 51.435)
  line L506 (12.5412, 50.8) -> (11.2713, 50.8)
  line L507 (11.6523, 51.816) -> (12.1603, 51.816)
  line L508 (11.6523, 52.324) -> (11.6523, 51.816)
  line L509 (12.1603, 52.324) -> (11.6523, 52.324)
  line L510 (12.1603, 51.816) -> (12.1603, 52.324)
  line L511 (13.1763, 51.435) -> (12.5412, 50.8)
  line L512 (13.1763, 51.435) -> (13.1763, 52.705)
  line L513 (11.2713, 53.34) -> (12.5412, 53.34)
  line L514 (10.6363, 52.705) -> (11.2713, 53.34)
  line L515 (12.5412, 53.34) -> (13.1763, 52.705)
  line L516 (13.1763, 52.705) -> (13.8113, 53.34)
  line L517 (13.8113, 53.34) -> (15.0813, 53.34)
  line L518 (15.7163, 53.34) -> (15.0813, 53.34)
  line L519 (15.7163, 52.705) -> (15.7163, 53.34)
  line L520 (15.7163, 51.435) -> (15.7163, 52.705)
  line L521 (15.0813, 50.8) -> (15.7163, 51.435)
  line L522 (15.0813, 50.8) -> (13.8113, 50.8)
  line L523 (13.8113, 50.8) -> (13.1763, 51.435)
  line L524 (14.1923, 51.816) -> (14.7003, 51.816)
  line L525 (14.1923, 52.324) -> (14.1923, 51.816)
  line L526 (14.7003, 52.324) -> (14.1923, 52.324)
  line L527 (14.7003, 51.816) -> (14.7003, 52.324)
  line L528 (4.445, 35.7188) -> (3.175, 35.7188)
  line L529 (3.175, 35.7188) -> (2.54, 35.7188)
  line L530 (2.54, 35.7188) -> (2.54, 35.0838)
  line L531 (2.54, 33.8137) -> (2.54, 35.0838)
  line L532 (3.175, 33.1788) -> (2.54, 33.8137)
  line L533 (3.556, 34.7028) -> (3.556, 34.1948)
  line L534 (4.064, 34.7028) -> (3.556, 34.7028)
  line L535 (4.064, 34.1948) -> (4.064, 34.7028)
  line L536 (3.556, 34.1948) -> (4.064, 34.1948)
  line L537 (4.445, 33.1788) -> (3.175, 33.1788)
  line L538 (2.54, 32.5438) -> (3.175, 33.1788)
  line L539 (2.54, 31.2738) -> (2.54, 32.5438)
  line L540 (3.175, 30.6388) -> (2.54, 31.2738)
  line L541 (4.445, 30.6388) -> (3.175, 30.6388)
  line L542 (3.556, 31.6548) -> (4.064, 31.6548)
  line L543 (3.556, 32.1628) -> (3.556, 31.6548)
  line L544 (4.064, 32.1628) -> (3.556, 32.1628)
  line L545 (4.064, 31.6548) -> (4.064, 32.1628)
  line L546 (4.445, 33.1788) -> (5.08, 32.5438)
  line L547 (5.08, 32.5438) -> (5.08, 31.2738)
  line L548 (5.08, 31.2738) -> (4.445, 30.6388)
  line L549 (5.08, 33.8137) -> (4.445, 33.1788)
  line L550 (5.08, 35.0838) -> (5.08, 33.8137)
  line L551 (5.08, 35.0838) -> (4.445, 35.7188)
  line L552 (32.6707, 38.7985) -> (15.9068, 38.7985) construction
  arc A67 (15.9068, 34.8615) -> (15.9068, 36.8935) centre (15.9068, 35.8775) ccw construction
  line L553 (15.9068, 32.9565) -> (32.6707, 32.9565) construction
  line L554 (32.6707, 28.4798) -> (15.9068, 28.4798) construction
  arc A68 (15.9068, 24.5427) -> (15.9068, 26.5747) centre (15.9068, 25.5587) ccw construction
  line L555 (15.9068, 22.6378) -> (32.6707, 22.6378) construction
  point P0 (8.0962, 52.705)
  constraint collinear L6 L553
  constraint collinear L8 L555
extrude "Extrude1" add sketch "DXF import" against normal blind 1.6 contours A0 L0 L1 A1 L2 L3 A2 A3 L16 L20 L21 L24 L25 L28 L29 L31 L32 L36 L37 L40 L42 L44 L45 L46 L48 L49 L50 L52 L55 L57 L60 L61 L62 L64 L65 L66 L68 L70 L76 L77 L80 L97 L98 L103 L104 L372 L373 L375 A23 L380 A27 L389 A32 L391 L392 A34 A37 L395 L397 L399 L402 L403 A38 L404 L407 L408 L409 L411 A40 A41 L413 L414 L415 L417 L421 L424 A51 A53 L431 A55 A57 | L3 L98 L104 L404 L411 A53 | L3 L29 L77 L408 A51 L431 | L3 L20 L21 L373 A23 L380 | L3 L68 L97 A38 L409 L415 | L3 L31 L32 L372 L389 A34 | L3 L62 L80 L417 L421 A57 | L3 L50 L60 A37 L414 L424 | L3 L61 L65 L407 L413 A55 | L3 L37 L40 L375 L397 A41 | L3 L64 L66 A27 L391 L395 | L3 L25 L55 A32 L392 L403 | L3 L44 L46 L399 L402 A40 | A4 | L4 L6 L12 A9 L26 L27 | A5 L5 L7 L8 L9 L10 | A6 | L13 L15 L17 A8 L18 L19 | L109 L114 L118 L142 L145 L147 | L109 L125 L141 L148 L155 L185 | L125 L133 L145 L167 | L121 L155 L167 L172 | L120 L121 L129 L133 L137 L138 L142 L144 L149 L152 | L110 L114 L119 L168 L171 L173 | L113 L130 L144 L170 L172 L185 | L118 L129 L132 L171 | L126 L132 L138 L173 | L124 L128 L143 L157 L169 L170 L187 L190 | L122 L126 L151 L152 L168 L190 | L130 L149 L156 L169 | L137 L156 L174 L187 | L120 L122 L157 L174 | L143 A12 | L143 A14 | L143 A15 | A11 L195 | L158 L159 L161 L164 L177 L186 L195 L197 | A16 L195 | A13 L195 | L165 L166 L179 L182 L197 L228 | L159 L180 L193 L196 L229 L231 | L166 L177 L192 L215 | L165 L203 L206 L213 L225 L234 | L161 L163 L189 L193 | L180 L183 L188 L191 L210 L218 | L162 L163 L175 L179 L181 L184 L192 L196 L201 L209 | L162 L186 L189 L215 | L178 L182 L209 L225 | L160 L184 L188 L231 | L176 L178 L181 L203 | L175 L176 L183 L194 L214 L234 | L160 L191 L201 L214 | L208 L235 L251 L253 L262 L263 | L198 L202 L207 L216 L224 L251 L255 L267 | L200 L204 L212 L221 L226 L263 | L202 L233 L262 L264 | A20 L267 | L212 L253 L256 L271 | L224 L232 L233 L259 | L205 L211 L217 L219 L230 L235 L240 L256 L259 L264 | L204 L220 L222 L230 L245 L260 | L205 L222 L226 L271 | L216 L217 L223 L232 | A17 L267 | L220 L247 L248 L252 L254 L276 | L199 L207 L219 L223 L237 L247 | L211 L227 L245 L248 | A18 L267 | L199 L227 L240 L254 | L236 L249 L272 L286 | L249 L275 L284 L287 | L236 L238 L242 L244 L246 L277 L283 L285 L287 L297 | L258 L269 L285 L286 L292 L296 | L261 L265 L266 L272 L279 L284 L288 L292 | L244 L274 L275 L288 | L277 L294 L295 L296 | L250 L274 L279 L291 L293 L297 | L239 L270 L283 L295 | L239 L241 L243 L269 L282 L294 | L238 L250 L278 L289 | L246 L257 L270 L273 L282 L290 | L242 L273 L280 L289 | L268 L278 L280 L281 L290 L293 | A19 L266 | L266 A21 | L266 A22 | L299 L316 L322 L337 | L300 L309 L315 L338 | L301 L304 L311 L334 | L302 L308 L323 L330 | L303 L319 L327 L332 | L305 L312 L328 L336 | L306 L307 L318 L335 | L310 L314 L324 L331 | L313 L317 L321 L329 | L320 L325 L333 L339 | L326 L443 L451 L461 | L340 L350 L351 L360 | L341 L354 L362 L364 | L342 L346 L358 L368 | L343 L355 L359 L365 | L344 L382 L384 L385 | L345 L352 L361 L378 | L347 L357 L367 L369 | L348 L366 L370 L381 | L349 L353 L356 L363 | L371 L376 L379 L383 | L374 L377 A24 A25 | A26 A33 L393 L401 | L386 A30 L396 A43 | A28 L387 A29 L394 | L388 L416 A48 A49 | A31 L390 A36 L398 | A35 L400 A50 L436 | L405 L418 A52 A58 | L406 A42 L420 A47 | L410 A39 A45 L422 | L412 A46 L423 A54 | A44 L419 L434 A56 | L425 L427 L432 L486 | L426 L429 L440 L441 | L428 L438 L439 L450 | L430 L433 L456 L471 | L435 L437 L455 L478 | L442 L445 L479 L483 | L444 L447 L452 L463 | L446 L453 L476 L490 | L448 L459 L460 L481 | L449 L454 L458 L477 | L457 L462 L484 L487 | L464 L468 L475 L485 | L465 L467 L469 L480 | L466 L474 L488 L489 | L470 L472 L473 L482 | A59 | A60 A61 A62 L491 | A64 | A63 L492 A65 A66 | L493 L494 L495 L496 L497 L498 L503 L504 | L504 L505 L506 L511 L512 L513 L514 L515 | L512 L516 L517 L518 L519 L520 L521 L522 L523 | L499 L500 L501 L502 | L507 L508 L509 L510 | L524 L525 L526 L527 | L528 L529 L530 L531 L532 L537 L549 L550 L551 | L537 L538 L539 L540 L541 L546 L547 L548 | L533 L534 L535 L536 | L542 L543 L544 L545 makes body 1 in component "PCB"
extrude "Extrude2" add sketch "DXF import" along normal blind 2.2 contours L109 L114 L118 L142 L145 L147 | L120 L121 L129 L133 L137 L138 L142 L144 L149 L152 | L113 L130 L144 L170 L172 L185 | L122 L126 L151 L152 L168 L190 | L165 L166 L179 L182 L197 L228 | L159 L180 L193 L196 L229 L231 | L162 L163 L175 L179 L181 L184 L192 L196 L201 L209 | L175 L176 L183 L194 L214 L234 | L208 L235 L251 L253 L262 L263 | L205 L211 L217 L219 L230 L235 L240 L256 L259 L264 | L204 L220 L222 L230 L245 L260 | L199 L207 L219 L223 L237 L247 | L236 L238 L242 L244 L246 L277 L283 L285 L287 L297 | L258 L269 L285 L286 L292 L296 | L250 L274 L279 L291 L293 L297 | L246 L257 L270 L273 L282 L290 | L493 L494 L495 L496 L497 L498 L503 L504 | L504 L505 L506 L511 L512 L513 L514 L515 | L512 L516 L517 L518 L519 L520 L521 L522 L523 | L528 L529 L530 L531 L532 L537 L549 L550 L551 | L537 L538 L539 L540 L541 L546 L547 L548 bodies 1 in component "PCB"
extrude "Extrude3" add sketch "DXF import" along normal blind 8.8 contours L109 L125 L141 L148 L155 L185 | L125 L133 L145 L167 | L121 L155 L167 L172 | L110 L114 L119 L168 L171 L173 | L118 L129 L132 L171 | L126 L132 L138 L173 | L124 L128 L143 L157 L169 L170 L187 L190 | L130 L149 L156 L169 | L137 L156 L174 L187 | L120 L122 L157 L174 | L158 L159 L161 L164 L177 L186 L195 L197 | L166 L177 L192 L215 | L165 L203 L206 L213 L225 L234 | L161 L163 L189 L193 | L180 L183 L188 L191 L210 L218 | L162 L186 L189 L215 | L178 L182 L209 L225 | L160 L184 L188 L231 | L176 L178 L181 L203 | L160 L191 L201 L214 | L198 L202 L207 L216 L224 L251 L255 L267 | L200 L204 L212 L221 L226 L263 | L202 L233 L262 L264 | L212 L253 L256 L271 | L224 L232 L233 L259 | L205 L222 L226 L271 | L216 L217 L223 L232 | L220 L247 L248 L252 L254 L276 | L211 L227 L245 L248 | L199 L227 L240 L254 | L236 L249 L272 L286 | L249 L275 L284 L287 | L261 L265 L266 L272 L279 L284 L288 L292 | L244 L274 L275 L288 | L277 L294 L295 L296 | L239 L270 L283 L295 | L239 L241 L243 L269 L282 L294 | L238 L250 L278 L289 | L242 L273 L280 L289 | L268 L278 L280 L281 L290 L293 bodies 1 in component "PCB"
extrude "Extrude4" add sketch "DXF import" along normal blind 8.5 contours L299 L316 L322 L337 | L300 L309 L315 L338 | L301 L304 L311 L334 | L302 L308 L323 L330 | L303 L319 L327 L332 | L305 L312 L328 L336 | L306 L307 L318 L335 | L310 L314 L324 L331 | L313 L317 L321 L329 | L320 L325 L333 L339 | L326 L443 L451 L461 | L340 L350 L351 L360 | L341 L354 L362 L364 | L342 L346 L358 L368 | L343 L355 L359 L365 | L344 L382 L384 L385 | L345 L352 L361 L378 | L347 L357 L367 L369 | L348 L366 L370 L381 | L349 L353 L356 L363 | L371 L376 L379 L383 | L425 L427 L432 L486 | L426 L429 L440 L441 | L428 L438 L439 L450 | L430 L433 L456 L471 | L435 L437 L455 L478 | L442 L445 L479 L483 | L444 L447 L452 L463 | L446 L453 L476 L490 | L448 L459 L460 L481 | L449 L454 L458 L477 | L457 L462 L484 L487 | L464 L468 L475 L485 | L465 L467 L469 L480 | L466 L474 L488 L489 | L470 L472 L473 L482 | L499 L500 L501 L502 | L507 L508 L509 L510 | L524 L525 L526 L527 | L533 L534 L535 L536 | L542 L543 L544 L545 bodies 1 in component "PCB"
chamfer "Chamfer1" distance 0.5 angle 45 28 edges at (2.6987, 18.5738, 8.8) (6.8262, 27.4638, 8.8) (9.3663, 24.0507, 8.8) (9.3663, 13.0968, 8.8) (6.8262, 9.6837, 8.8) (2.7781, 27.4638, 8.8) (2.7781, 9.6837, 8.8) (48.7937, 9.65, 8.8) (51.3338, 12.19, 8.8) (44.7456, 9.65, 8.8) (44.6662, 16, 8.8) (44.7456, 22.35, 8.8) (48.7938, 22.35, 8.8) (51.3338, 19.81, 8.8) (44.7456, 26.11, 8.8) (48.7937, 26.11, 8.8) (44.6662, 35, 8.8) (51.3338, 29.5231, 8.8) (51.3338, 40.4769, 8.8) (48.7938, 43.89, 8.8) (44.7456, 43.89, 8.8) (32.4769, 53.3338, 8.8) (35.89, 50.7937, 8.8) (35.89, 46.7456, 8.8) (27, 46.6662, 8.8) (18.11, 46.7456, 8.8) (18.11, 50.7938, 8.8) (21.5231, 53.3338, 8.8) on bodies 1 in component "PCB"
extrude "Extrude5" add sketch "DXF import" against normal blind 0.5 from surface at -1.6 contours L3 L98 L104 L404 L411 A53 | L3 L98 L104 L135 | L3 L29 L77 L408 A51 L431 | L3 L29 L77 L135 | L3 L20 L21 L135 | L3 L20 L21 L373 A23 L380 | L3 L68 L97 A38 L409 L415 | L3 L68 L97 L135 | L3 L31 L32 L135 | L3 L31 L32 L372 L389 A34 | L3 L62 L80 L417 L421 A57 | L3 L62 L80 L135 | L3 L50 L60 L135 | L3 L50 L60 A37 L414 L424 | L3 L61 L65 L407 L413 A55 | L3 L61 L65 L135 | L3 L37 L40 L135 | L3 L37 L40 L375 L397 A41 | L3 L64 L66 A27 L391 L395 | L3 L64 L66 L135 | L3 L25 L55 L135 | L3 L25 L55 A32 L392 L403 | L3 L44 L46 L399 L402 A40 | L3 L44 L46 L135 bodies 1 in component "PCB"
extrude "Extrude6" add sketch "DXF import" against normal blind 8.8 from surface at 4 contours L3 L79 L103 L108 L135 | L69 L72 L73 L74 L75 L78 L86 L87 L91 L92 L95 L101 L102 L111 L112 L115 L116 L135 L136 L139 L153 L154 L298 | L3 L34 L36 L38 L135 | L3 L11 L23 L24 L135 | L3 L63 L70 L96 L135 | L3 L14 L16 L22 L135 | L3 L39 L42 L105 L135 | L3 L30 L51 L52 L135 | L3 L43 L67 L76 L135 | L3 L41 L48 L54 L135 | L3 L28 L35 L71 L135 | L3 L49 L56 L59 L135 | L3 L47 L53 L57 L135 | L3 L33 L45 L58 L135 bodies 1 in component "PCB"
extrude "Extrude7" add sketch "C64_Userport_Test" along normal blind 10.7 contours A12 | A14 bodies 1 in component "PCB"
extrude "Extrude8" add sketch "DXF import" along normal blind 6.5 contours A60 A61 A62 L491 | A63 L492 A65 A66 bodies 1 in component "PCB"
fillet "Fillet1" radius 1.4 2 edges at (6.1015, 44.4576, 10.7) (11.6015, 44.4576, 10.7) on bodies 1 in component "PCB"
ref_plane "WorkPlane1" through (0, 0, -4.4) normal (0, 0, 1) x (1, 0, 0) in component "diag_up_bottom_noVM"